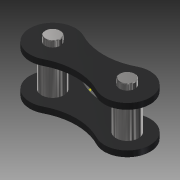
# Autodesk Inventor part: ConnectingLinks
Saved by Autodesk Inventor 2014 (Build 180170000, 170)
## iProperties
Created: 2013-07-15
Part Number: ConnectingLinks
Material: Generic
Document SubType Name: Modeling
Designer: Mill
Density: 1 g/cm^3
Appearance: Default
Author: Mill
Autodesk Inventor part; units mm, degrees
ref_plane "YZ Plane" through (0, 0, 0) normal (1, 0, 0) x (0, 1, 0)
ref_plane "XZ Plane" through (0, 0, 0) normal (0, 1, 0) x (-1, 0, 0)
sketch "Sketch1" plane through (0, 0, 0) normal (0, 0, 1) x (1, 0, 0)
  circle A0 centre (-6.35, 0) radius 3.885
  circle A1 centre (6.35, 0) radius 3.885
  arc A2 (-4.5733, 3.4549) -> (4.5733, 3.4549) centre (0, 12.3479) ccw
  arc A3 (4.5733, -3.4549) -> (-4.5733, -3.4549) centre (0, -12.3479) ccw
  point P0 (0, 0)
  dimension "d0" = 7.77
  dimension "d1" = 6.35
  dimension "d2" = 7.77
  dimension "d3" = 6.35
  dimension "d4" = 20
  dimension "d5" = 0
  dimension "d6" = 0
  dimension "d7" = 20
  constraints: 8 point on circle, 4 centre point, 4 tangent
  measures "d0" diameter of A0
  measures "d1" distance of A0.centre point (0, 0)
  measures "d2" diameter of A1
  measures "d3" distance of A1.centre point (0, 0)
  measures "d4" diameter of A2
  measures "d5" vertical distance of point (0, 0) A0.centre
  measures "d6" vertical distance of point (0, 0) A1.centre
  measures "d7" diameter of A3
extrude "Extrusion1" add sketch "Sketch1" along normal blind 1
sketch "Sketch2" plane through (0, 0, 0) normal (0, 0, -1) x (-1, 0, 0)
  arc A0 (-4.5733, 3.4549) -> (-4.5733, -3.4549) centre (-6.35, 0) ccw projected
  arc A1 (4.5733, -3.4549) -> (4.5733, 3.4549) centre (6.35, 0) ccw projected
  circle A2 centre (-6.35, 0) radius 1.9
  circle A3 centre (6.35, 0) radius 1.9
  point P0 (0, 0)
  dimension "d10" = 3.8
  dimension "d11" = 3.8
  constraints: 2 centre point, 2 coincident
  measures "d10" diameter of A2
  measures "d11" diameter of A3
extrude "Extrusion2" add sketch "Sketch2" along normal blind 6
sketch "Sketch3" plane through (-6.35, 0, -6) normal (0, 0, -1) x (-1, 0, 0)
  circle A0 centre (-12.7, 0) radius 1.9 projected
  circle A1 centre (0, 0) radius 1.9 projected
  arc A2 (-10.9233, 3.4549) -> (-1.7767, 3.4549) centre (-6.35, 12.3479) ccw projected
  arc A3 (-10.9233, 3.4549) -> (-10.9233, -3.4549) centre (-12.7, 0) ccw projected
  arc A4 (-1.7767, -3.4549) -> (-10.9233, -3.4549) centre (-6.35, -12.3479) ccw projected
  arc A5 (-1.7767, -3.4549) -> (-1.7767, 3.4549) centre (0, 0) ccw projected
  point P0 (-6.35, 0)
extrude "Extrusion3" add sketch "Sketch3" along normal blind 1 contours A0 | A1 | A2 A5 A4 A3
sketch "Sketch4" plane through (0, 0, 1) normal (0, 0, 1) x (1, 0, 0)
  arc A0 (-4.5733, 3.4549) -> (-4.5733, -3.4549) centre (-6.35, 0) ccw projected
  arc A1 (4.5733, -3.4549) -> (4.5733, 3.4549) centre (6.35, 0) ccw projected
  circle A2 centre (-6.35, 0) radius 1.3
  circle A3 centre (6.35, 0) radius 1.3
  point P0 (0, 0)
  dimension "d16" = 2.6
  dimension "d17" = 2.6
  constraints: 2 centre point, 2 coincident
  measures "d16" diameter of A2
  measures "d17" diameter of A3
extrude "Extrusion4" add sketch "Sketch4" along normal blind 1
sketch "Sketch5" plane through (-6.35, 0, -7) normal (0, 0, -1) x (-1, 0, 0)
  arc A0 (-10.9233, 3.4549) -> (-10.9233, -3.4549) centre (-12.7, 0) ccw projected
  arc A1 (-1.7767, -3.4549) -> (-1.7767, 3.4549) centre (0, 0) ccw projected
  circle A2 centre (-12.7, 0) radius 1.3
  circle A3 centre (0, 0) radius 1.3
  point P0 (-6.35, 0)
  dimension "d20" = 2.6
  dimension "d21" = 2.6
  constraints: 2 centre point, 2 coincident
  measures "d20" diameter of A2
  measures "d21" diameter of A3
extrude "Extrusion5" add sketch "Sketch5" along normal blind 1
chamfer "Chamfer1" distance 0.1 angle 45 2 edges at (7.65, 0, -8) (-5.05, 0, -8)
chamfer "Chamfer2" distance 0.1 angle 45 2 edges at (5.05, 0, 2) (-7.65, 0, 2)
ref_plane "Work Plane1" through (0, 0, -3) normal (0, 0, 1) x (1, 0, 0)
equation "\"d2\" = d0"
equation "\"d3\" = d1"
equation "\"d7\" = d4"
equation "\"d11\" = d10"
equation "\"d17\" = d16"
equation "\"d20\" = d16"
equation "\"d21\" = d16"
body "Solid1"
